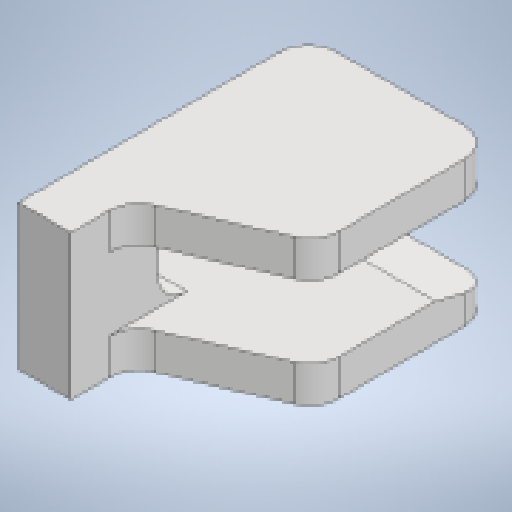
# Autodesk Inventor part: MolexClipper_vertical
Saved by Autodesk Inventor 2025.1 (Build 291241000, 241)
## iProperties
Created: 2026-05-09
Part Number: MolexClipper_vertical
Material: Generic
Document SubType Name: Modeling
Designer: User
Density: 1 g/cm^3
Appearance: Default
Author: User
## iProperties of the stored document MolexClipper_vertical_3DPrint.ipt
Created: 2026-05-09
Part Number: MolexClipper_vertical_3DPrint
Material: Generic
Document SubType Name: Modeling
Designer: User
Density: 1 g/cm^3
Appearance: Default
Author: User
Autodesk Inventor part; units mm, degrees
ref_plane "YZ Plane" through (0, 0, 0) normal (1, 0, 0) x (0, 1, 0)
ref_plane "XZ Plane" through (0, 0, 0) normal (0, 1, 0) x (-1, 0, 0)
ref_plane "XY Plane" through (0, 0, 0) normal (0, 0, 1) x (1, 0, 0)
sketch "Sketch1" plane through (0, 0, 0) normal (0, 0, 1) x (1, 0, 0)
  line L0 (-4.78, -2.9) -> (4.78, -2.9)
  line L1 (6.35, 2.9) -> (-6.35, 2.9)
  line L2 (-4.78, -2.9) -> (-5.08, -2.9)
  line L3 (-6.35, -2.9) -> (-5.08, -2.9)
  line L4 (-6.35, 2.9) -> (-6.35, -2.9)
  line L5 (5.08, -2.9) -> (4.78, -2.9)
  line L6 (5.08, -2.9) -> (6.35, -2.9)
  line L7 (6.35, 3) -> (-6.45, 3)
  line L8 (-6.45, 3) -> (-6.45, -3)
  line L9 (-6.45, -3) -> (-5.08, -3)
  line L10 (-5.08, -3) -> (-4.78, -3)
  line L11 (-4.78, -3) -> (4.78, -3)
  line L12 (4.78, -3) -> (5.08, -3)
  line L13 (5.08, -3) -> (6.35, -3)
  line L14 (6.35, 5) -> (-8.45, 5)
  line L15 (-8.45, 5) -> (-8.45, -5)
  line L16 (-8.45, -5) -> (-5.08, -5)
  line L17 (-5.08, -5) -> (-4.78, -5)
  line L18 (-4.78, -5) -> (4.78, -5)
  line L19 (4.78, -5) -> (5.08, -5)
  line L20 (5.08, -5) -> (6.35, -5)
  line L21 (6.35, 3) -> (6.35, 5)
  line L22 (6.35, -3) -> (6.35, -5)
  point P0 (0, 0)
extrude "Extrusion1" add sketch "Sketch1" against normal blind 2
sketch "Sketch2" plane through (-8.45, -5, 0) normal (0, -1, 0) x (1, 0, 0)
  line L0 (2.1, -8) -> (2.1, -11.17) projected
  line L1 (0, 0) -> (14.8, 0) projected
  line L2 (2.1, -8) -> (3.37, -8) projected
  line L3 (14.8, 0) -> (14.8, -2) projected
  line L4 (2, 0) -> (14.8, 0) projected
  line L5 (2, 0) -> (14.8, 0)
  line L6 (14.8, 0) -> (14.8, -8)
  line L7 (14.8, -8) -> (2, -8)
  line L8 (2, -8) -> (2, 0)
  point P0 (8.45, 0)
  constraints: 8 end point, 2 parallel, 1 horizontal, 1 perpendicular
extrude "Extrusion2" add sketch "Sketch2" against normal up to surface (2 mm away)
sketch "Sketch3" plane through (-8.45, 5, 0) normal (0, 1, 0) x (1, 0, 0)
  line L0 (0, 0) -> (14.8, 0) projected
  line L1 (0, 0) -> (0, 2) projected
  line L2 (2, 2) -> (0, 2) projected
  line L3 (2, 2) -> (2, 8) projected
  line L4 (2, 8) -> (14.8, 8) projected
  line L5 (14.8, 0) -> (14.8, 8) projected
  point P0 (8.45, 0)
extrude "Extrusion3" add sketch "Sketch3" against normal up to surface (2 mm away)
sketch "Sketch4" plane through (-8.45, -5, 0) normal (0, -1, 0) x (1, 0, 0)
  line L0 (2, -2) -> (2, -8) projected
  line L1 (0, 0) -> (14.8, 0) projected
  line L2 (3.67, -0.6428) -> (3.67, -14.175) projected
  line L3 (5.61, -0.6428) -> (5.61, -14.175) projected
  line L4 (2, -2) -> (5.61, -2)
  line L5 (5.61, -2) -> (5.61, 4)
  line L6 (5.61, 4) -> (2, 4)
  line L7 (2, 4) -> (2, -2)
  point P0 (8.45, 0)
  point P1 (2, 0)
  point P2 (5.61, 0)
  dimension "d8" = 6
  constraints: 8 end point, 2 parallel, 1 horizontal, 1 perpendicular, 1 point on line
  measures "d8" distance of L5.end L4.end
extrude "Extrusion4" add sketch "Sketch4" against normal up to surface (10 mm away) contours L7 L6 L5 L1
sketch "Sketch5" plane through (-8.45, -5, -2) normal (0, -1, 0) x (1, 0, 0)
  line L0 (0, 2) -> (0, 0) projected
  line L1 (0, 2) -> (2, 2) projected
  line L2 (2, 0) -> (0, 0) projected
  line L3 (0, 2) -> (2, 2)
  line L4 (2, 2) -> (2, 0)
  line L5 (2, 0) -> (0, 0)
  line L6 (0, 0) -> (0, 2)
  point P0 (8.45, 2)
  constraints: 8 end point, 2 parallel, 1 horizontal, 1 perpendicular
extrude "Extrusion5" cut sketch "Sketch5" against normal through all
sketch "Sketch6" plane through (-6.45, -5, -8) normal (0, -1, 0) x (1, 0, 0)
  line L0 (3.61, 8) -> (3.61, 12) projected
  line L1 (3.61, 8) -> (12.8, 8) projected
  line L2 (3.61, 12) -> (12.8, 8)
  point P0 (6.45, 8)
  constraints: 2 end point
extrude "Extrusion6" add sketch "Sketch6" against normal up to surface (2 mm away)
sketch "Sketch7" plane through (-6.45, 5, -8) normal (0, 1, 0) x (1, 0, 0)
  line L0 (12.8, -8) -> (3.61, -12) projected
  line L1 (12.8, -8) -> (3.61, -8) projected
  line L2 (3.61, -8) -> (3.61, -12) projected
  point P0 (6.45, -8)
extrude "Extrusion7" add sketch "Sketch7" against normal up to surface (2 mm away)
sketch "Sketch8" plane through (-2.84, -3, 0) normal (1, 0, 0) x (0, 0, -1)
  line L0 (0, 6) -> (-4, 6) projected
  line L1 (-4, 0) -> (-4, 6) projected
  line L2 (-4, 0) -> (0, 0) projected
  line L3 (0, 0) -> (0, 6) projected
  line L4 (-4, 0) -> (0, 0) projected
  line L5 (-2, 0) -> (-2, 6)
  point P0 (0, 3)
  point P1 (-2, 0)
  constraints: 2 end point, 2 midpoint
extrude "Extrusion8" cut sketch "Sketch8" against normal blind 10 contours L3 L2 L5 L0
sketch "Sketch9" plane through (-6.45, -5, 4) normal (0, 0, 1) x (1, 0, 0)
  line L0 (0, 8) -> (0, 2) projected
  line L1 (3.61, 10) -> (0, 10) projected
  line L2 (0, 0) -> (0, 10) projected
  line L3 (3.61, 0) -> (0, 0) projected
  line L4 (3.61, 0) -> (3.61, 2) projected
  line L5 (3.61, 2) -> (3.61, 8) projected
  line L6 (3.61, 8) -> (3.61, 10) projected
  point P0 (6.45, 5)
  point P1 (0, 2)
extrude "Extrusion9" add sketch "Sketch9" along normal blind 4
fillet "Fillet1" radius 2 4 edges at (-2.84, 4, 4) (-2.84, -4, 4) (6.35, 4, 0) (6.35, -4, 0)
sketch "Sketch10" plane through (6.35, -5, -8) normal (0, 0, -1) x (-1, 0, 0)
  line L0 (12.8, 2) -> (0, 2) projected
  line L1 (0, 0) -> (0, 2) projected
  line L2 (12.8, 0) -> (0, 0) projected
  line L3 (12.8, 0) -> (12.8, 2) projected
  line L4 (0, 8) -> (12.8, 8) projected
  line L5 (12.8, 10) -> (12.8, 8) projected
  line L6 (0, 10) -> (12.8, 10) projected
  line L7 (0, 10) -> (0, 8) projected
  point P0 (6.35, 5)
extrude "Extrusion10" add sketch "Sketch10" along normal blind 4
sketch "Sketch11" plane through (-6.45, 3, 2) normal (0, -1, 0) x (1, 0, 0)
  arc A0 (12.8, -3.3107) -> (11.5982, -1.4769) centre (10.8, -3.3107) ccw projected
  line L0 (4.8118, 1.4769) -> (11.5982, -1.4769) projected
  arc A1 (3.61, 3.3107) -> (4.8118, 1.4769) centre (5.61, 3.3107) ccw projected
  line L1 (3.61, 0) -> (3.61, 3.3107) projected
  line L2 (3.61, 0) -> (0, 0) projected
  line L3 (0, 0) -> (0, -14) projected
  line L4 (12.8, -14) -> (0, -14) projected
  line L5 (12.8, -3.3107) -> (12.8, -14) projected
  point P0 (6.45, -2)
extrude "Extrusion11" add sketch "Sketch11" along normal blind 0.5
sketch "Sketch12" plane through (-6.45, -3, 2) normal (0, 1, 0) x (1, 0, 0)
  arc A0 (11.5982, 1.4769) -> (12.8, 3.3107) centre (10.8, 3.3107) ccw projected
  line L0 (12.8, 3.3107) -> (12.8, 14) projected
  line L1 (0, 14) -> (12.8, 14) projected
  line L2 (0, 0) -> (0, 14) projected
  line L3 (3.61, 0) -> (0, 0) projected
  line L4 (3.61, -3.3107) -> (3.61, 0) projected
  arc A1 (4.8118, -1.4769) -> (3.61, -3.3107) centre (5.61, -3.3107) ccw projected
  line L5 (11.5982, 1.4769) -> (4.8118, -1.4769) projected
  point P0 (6.45, 2)
extrude "Extrusion12" add sketch "Sketch12" along normal blind 0.5
fillet "Fillet3" radius 2 2 edges at (-4.645, -2.5, 2) (-4.645, 2.5, 2)
sketch "Sketch14" plane through (6.35, -5, -12) normal (0, 0, -1) x (-1, 0, 0)
  line L0 (0, 0) -> (0, 2.5) projected
  line L1 (0, 0) -> (12.8, 0) projected
  line L2 (12.8, 0) -> (12.8, 2.5) projected
  line L3 (0, 2.5) -> (12.8, 2.5) projected
  line L4 (12.8, 10) -> (12.8, 7.5) projected
  line L5 (12.8, 10) -> (0, 10) projected
  line L6 (0, 10) -> (0, 7.5) projected
  line L7 (12.8, 7.5) -> (0, 7.5) projected
  point P0 (6.35, 5)
extrude "Extrusion13" add sketch "Sketch14" along normal blind 5
sketch "Sketch15" plane through (6.35, -5, -17) normal (0, 0, -1) x (-1, 0, 0)
  line L0 (12.8, 2.5) -> (0, 2.5) projected
  line L1 (0, 2.5) -> (0, 0) projected
  line L2 (0, 0) -> (12.8, 0) projected
  line L3 (12.8, 0) -> (12.8, 2.5) projected
  line L4 (0, 7.5) -> (12.8, 7.5) projected
  line L5 (12.8, 7.5) -> (12.8, 10) projected
  line L6 (12.8, 10) -> (0, 10) projected
  line L7 (0, 10) -> (0, 7.5) projected
  line L8 (12.8, 0) -> (10.3, 0)
  line L9 (10.3, 0) -> (10.3, -2.5)
  line L10 (10.3, -2.5) -> (12.8, -2.5)
  line L11 (12.8, -2.5) -> (12.8, 0)
  line L12 (12.8, 10) -> (10.3, 10)
  line L13 (10.3, 10) -> (10.3, 12.5)
  line L14 (10.3, 12.5) -> (12.8, 12.5)
  line L15 (12.8, 12.5) -> (12.8, 10)
  line L16 (0, 10) -> (2.5, 10)
  line L17 (2.5, 10) -> (2.5, 12.5)
  line L18 (2.5, 12.5) -> (0, 12.5)
  line L19 (0, 12.5) -> (0, 10)
  line L20 (0, 0) -> (2.5, 0)
  line L21 (2.5, 0) -> (2.5, -2.5)
  line L22 (2.5, -2.5) -> (0, -2.5)
  line L23 (0, -2.5) -> (0, 0)
  point P0 (6.35, 5)
  point P1 (2.5, 10)
  point P2 (2.5, 0)
  dimension "d39" = 2.5
  dimension "d40" = 2.5
  dimension "d41" = 2.5
  dimension "d42" = 2.5
  dimension "d43" = 2.5
  dimension "d44" = 2.5
  dimension "d45" = 2.5
  dimension "d46" = 2.5
  constraints: 32 end point, 8 parallel, 4 horizontal, 4 perpendicular
  measures "d39" distance of L10.end L9.end
  measures "d40" distance of L9.end L8.end
  measures "d41" distance of L13.end L14.end
  measures "d42" distance of L12.end L13.end
  measures "d43" distance of L18.end L17.end
  measures "d44" distance of L17.end L16.end
  measures "d45" distance of L21.end L22.end
  measures "d46" distance of L20.end L21.end
extrude "Extrusion14" add sketch "Sketch15" against normal up to surface (25 mm away) contours L11 L10 L9 L2 | L2 L21 L22 L23 | L19 L18 L17 L6 | L6 L13 L14 L15
sketch "Sketch16" plane through (3.85, 5, 8) normal (0, -1, 0) x (1, 0, 0)
  line L0 (0, -6.9119) -> (1.2982, -7.4769) projected
  arc A0 (2.5, -9.3107) -> (1.2982, -7.4769) centre (0.5, -9.3107) ccw projected
  line L1 (2.5, -9.3107) -> (2.5, 0) projected
  line L2 (2.5, 0) -> (0, 0) projected
  line L3 (0, -6.9119) -> (0, 0) projected
  point P0 (-3.85, -8)
extrude "Extrusion15" cut sketch "Sketch16" along normal mid plane 31
fillet "Fillet5" radius 2 4 edges at (6.35, 5, -17) (-6.45, 5, -17) (6.35, -5, -17) (-6.45, -5, -17)
chamfer "Chamfer3" distance 2.5 angle 45 2 edges at (-5.2, -7.5, 8) (-5.2, 7.5, 8)
sketch "Sketch17" plane through (-6.45, 2.5, -15) normal (-1, 0, 0) x (0, 0, 1)
  line L0 (-2, 5) -> (-2, 0) projected
  line L1 (-2, 5) -> (0, 5) projected
  line L2 (0, 5) -> (20.5, 5) projected
  line L3 (0, 0) -> (-2, 0) projected
  line L4 (15, 0) -> (0, 0) projected
  line L5 (-2, 0) -> (-2, 1)
  line L6 (-2, 0) -> (-2, 5) projected
  line L7 (-2, 0) -> (2, 0)
  line L8 (2, 0) -> (-2, 1)
  point P0 (15, -2.5)
  point P1 (-2, 1)
  dimension "d55" = 1
  dimension "d56" = 4
  constraints: 6 end point, 2 point on line
  measures "d55" distance of L0.end L5.end
  measures "d56" distance of L0.end L7.end
extrude "Extrusion16" cut sketch "Sketch17" against normal blind 31
sketch "Sketch18" plane through (-6.45, -7.5, -15) normal (-1, 0, 0) x (0, 0, 1)
  line L0 (16.0881, 12.5) -> (-2, 12.5) projected
  line L1 (0, 15) -> (20.5, 15) projected
  line L2 (-2, 2.5) -> (16.0881, 2.5) projected
  line L3 (0, 0) -> (20.5, 0) projected
  line L4 (-2, 15) -> (0, 15) projected
  line L5 (-2, 15) -> (-2, 11) projected
  line L6 (-2, 5) -> (-2, 0) projected
  line L7 (0, 0) -> (-2, 0) projected
  line L8 (-2, 0) -> (4, 0)
  line L9 (4, 0) -> (-2, 2.5)
  line L10 (-2, 15) -> (4, 15)
  line L11 (4, 15) -> (-2, 12.5)
  point P0 (15, 7.5)
  dimension "d59" = 6
  dimension "d60" = 6
  constraints: 8 end point, 2 point on line
  measures "d59" distance of L6.end L8.end
  measures "d60" distance of L4.start L10.end
extrude "Extrusion17" cut sketch "Sketch18" against normal through all
body "Solid1"
